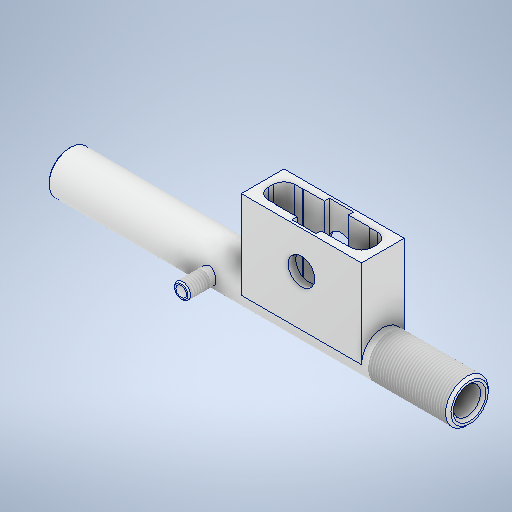
# Autodesk Inventor part: Riffelrør
Saved by Autodesk Inventor 2025.1 (Build 291241000, 241)
## iProperties
Created: 2025-02-26
Part Number: Riffelrør
Material: Aluminum 6061
Document SubType Name: Modeling
Designer: frede
Density: 2.7 g/cm^3
Appearance: Aluminum - Flat
Author: frede
Autodesk Inventor part; units mm, degrees
ref_plane "YZ Plane" through (0, 0, 0) normal (1, 0, 0) x (0, 1, 0)
sketch "Sketch1" plane through (0, 0, 0) normal (0, 0, 1) x (1, 0, 0)
  line L0 (0, 0) -> (150, 0)
  line L1 (150, 5) -> (150, 8)
  line L2 (150, 8) -> (0, 8)
  line L3 (0, 8) -> (0, 5)
  line L4 (0, 0) -> (150, 0)
  line L5 (150, 5) -> (0, 5)
  dimension "d0" = 150
  dimension "d1" = 8
  dimension "d2" = 5
  constraints: 12 end point, 3 parallel, 2 horizontal, 1 perpendicular
  measures "d0" distance of L2.end L1.end
  measures "d1" distance of L1.end L0.end
  measures "d2" distance of L1.start L4.end
revolve "Revolution1" add sketch "Sketch1" angle 360 about axis through (0, 0, 0) along (1, 0, 0)
ref_plane "Work Plane1" through (0, 0, 8) normal (0, 0, 1) x (1, 0, 0)
ref_plane "Work Plane2" through (0, 8, 0) normal (0, 1, 0) x (-1, 0, 0)
sketch "Sketch3" plane through (0, 8, 0) normal (0, 1, 0) x (-1, 0, 0)
  line L0 (-150, -5) -> (0, -5) projected
  line L1 (-150, 5) -> (0, 5) projected
  line L2 (-114.5, -5) -> (-75.5, -5)
  line L3 (-75.5, -5) -> (-75.5, 5)
  line L4 (-75.5, 5) -> (-114.5, 5)
  line L5 (-114.5, 5) -> (-114.5, -5)
  line L6 (-150, 8) -> (-150, -8) projected
  line L7 (-75.5, 5) -> (-114.5, -5)
  line L8 (0, 8) -> (-150, 8) projected
  line L9 (-72.5, -8) -> (-117.5, -8)
  line L10 (-117.5, -8) -> (-117.5, 8)
  line L11 (-117.5, 8) -> (-72.5, 8)
  line L12 (-72.5, 8) -> (-72.5, -8)
  line L13 (-72.5, -8) -> (-117.5, 8) construction
  line L14 (-117.5, -8) -> (-72.5, 8) construction
  point P0 (0, 0)
  point P1 (-95, 0)
  point P2 (-150, 0)
  dimension "d13" = 39
  dimension "d19" = 45
  dimension "d77" = 55
  dimension "d78" = 32.5
  constraints: 22 end point, 4 midpoint, 4 parallel, 3 point on line, 2 horizontal, 2 perpendicular
  measures "d13" distance of L4.end L3.end
  measures "d19" distance of L10.end L11.end
  measures "d77" distance of point (-150, 0) point (-95, 0)
  measures "d78" distance between parallel lines of L6 L10
extrude "Extrusion2" cut sketch "Sketch3" against normal blind 8 contours L7 L3 L0 | L5 L1 L7
extrude "Extrusion3" add sketch "Sketch3" along normal blind 25 and the other way blind 8 contours L0 L12 L9 L10 | L0 L10 L1 L5 | L3 L1 L12 L0 | L1 L10 L8 L12
sketch "Sketch4" plane through (72.5, 33, 8) normal (0, 0, 1) x (1, 0, 0)
  line L0 (77.5, -28) -> (-72.5, -28) projected
  circle A0 centre (22.5, -14) radius 15
  circle A1 centre (22.5, -14) radius 5
  line L1 (45, -33) -> (45, 0) projected
  line L2 (0, 0) -> (0, -33) projected
  point P0 (-72.5, -33)
  dimension "d25" = 30
  dimension "d26" = 14
  dimension "d27" = 10
  dimension "d80" = 45
  dimension "d81" = 22.5
  constraints: 2 centre point, 1 coincident
  measures "d25" diameter of A0
  measures "d26" distance from line of A0.centre L0
  measures "d27" diameter of A1
  measures "d80" distance between parallel lines of L1 L2
  measures "d81" distance from line of L1 A0.centre
extrude "Extrusion4" cut sketch "Sketch4" against normal blind 40 contours A1
thread "Thread4" size "M16x1" class "6g" standard "ISO Metric profile" length 30
chamfer "Chamfer1" distance 1 angle 45 1 edges at (150, -8, 0)
sketch "Sketch5" plane through (150, 0, 0) normal (1, 0, 0) x (0, 0, -1)
  circle A0 centre (0, 0) radius 5.125
  dimension "d39" = 10.25
  constraints: 1 centre point, 1 coincident
  measures "d39" diameter of A0
extrude "Extrusion5" cut sketch "Sketch5" against normal blind 150
chamfer "Chamfer2" distance 1 angle 45 1 edges at (150, 0, 5.125)
sketch "Sketch6" plane through (0, 33, 0) normal (0, 1, 0) x (1, 0, 0)
  line L0 (100, 5) -> (100, 8) projected
  line L1 (90, 5) -> (90, 8) projected
  line L2 (90, -8) -> (90, -5) projected
  line L3 (100, -8) -> (100, -5) projected
  line L4 (90, 5) -> (100, -5)
  line L5 (90, -5) -> (100, 5)
  line L6 (99.5, 7) -> (90.5, 7)
  line L7 (90.5, 7) -> (90.5, -7)
  line L8 (90.5, -7) -> (99.5, -7)
  line L9 (99.5, -7) -> (99.5, 7)
  line L10 (99.5, 7) -> (90.5, -7) construction
  line L11 (90.5, 7) -> (99.5, -7) construction
  line L12 (114.5, 5) -> (114.5, -5) projected
  line L13 (75.5, -5) -> (75.5, 5) projected
  point P0 (0, 0)
  point P1 (95, 0)
  dimension "d43" = 9
  dimension "d44" = 14
  dimension "d79" = 39
  constraints: 16 end point, 3 midpoint, 2 parallel, 2 perpendicular, 1 horizontal
  measures "d43" distance of L8.end L7.end
  measures "d44" distance of L7.end L6.end
  measures "d79" distance between parallel lines of L12 L13
extrude "Extrusion6" cut sketch "Sketch6" against normal up to surface
sketch "Sketch8" plane through (0, 0, 8) normal (0, 0, 1) x (1, 0, 0)
  circle A0 centre (60, 0) radius 2
  line L0 (150, 7) -> (150, -7) projected
  circle A1 centre (60, 0) radius 3
  point P0 (0, 0)
  dimension "d56" = 4
  dimension "d57" = 90
  dimension "d58" = 6
  constraints: 2 centre point, 1 coincident
  measures "d56" diameter of A0
  measures "d57" distance from line of L0 A0.centre
  measures "d58" diameter of A1
extrude "Extrusion9" cut sketch "Sketch8" against normal blind 5 contours A0
extrude "Extrusion10" add sketch "Sketch8" along normal blind 10 and the other way blind 1
thread "Thread5" size "M6x1" class "6g" standard "ANSI Metric M Profile" length 8
chamfer "Chamfer3" distance 0.5 angle 45 1 edges at (57, 0, 18)
chamfer "Chamfer4" distance 0.5 angle 45 2 edges at (0, -8, 0) (0, 0, 5.125)
sketch "Sketch9" plane through (0, 33, 0) normal (0, 1, 0) x (1, 0, 0)
  line L0 (75.5, -5) -> (75.5, 5) projected
  line L1 (114.5, 5) -> (114.5, -5) projected
  line L2 (75.5, 5) -> (114.5, -5)
  line L3 (107.5, 5.125) -> (82.5, 5.125)
  line L4 (82.5, 5.125) -> (82.5, -5.125)
  line L5 (82.5, -5.125) -> (107.5, -5.125)
  line L6 (107.5, -5.125) -> (107.5, 5.125)
  line L7 (107.5, 5.125) -> (82.5, -5.125) construction
  line L8 (82.5, 5.125) -> (107.5, -5.125) construction
  point P0 (0, 0)
  point P1 (95, 0)
  dimension "d73" = 25
  dimension "d74" = 10.25
  constraints: 14 end point, 3 midpoint, 2 parallel, 1 horizontal, 1 perpendicular
  measures "d73" distance of L5.end L4.end
  measures "d74" distance of L4.end L3.end
extrude "Extrusion11" cut sketch "Sketch9" against normal blind 33
fillet "Fillet1" radius 4 4 edges at (114.5, 17.0625, -5) (114.5, 17.0625, 5) (75.5, 17.0625, -5) (75.5, 17.0625, 5)
equation "\"d81\" = 0.5 * d80"
body "Solid1"
